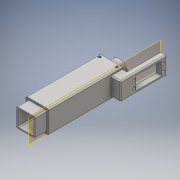
# Autodesk Inventor part: tube4
Saved by Autodesk Inventor 2016 (Build 200138000, 138)
## iProperties
Created: 2016-03-04
Part Number: tube4
Material: 一般
Document SubType Name: Modeling
Designer: Shun Hasegawa
Density: 1 g/cm^3
Appearance: 既定
Author: Shun Hasegawa
Autodesk Inventor part; units mm, degrees
ref_plane "XZ Plane" through (0, 0, 0) normal (0, 1, 0) x (-1, 0, 0)
ref_plane "XY Plane" through (0, 0, 0) normal (0, 0, 1) x (1, 0, 0)
sketch "スケッチ1" plane through (0, 0, 0) normal (0, 1, 0) x (-1, 0, 0)
  line L0 (16.5, 16.5) -> (-16.5, 16.5)
  line L1 (-16.5, 16.5) -> (-16.5, -16.5)
  line L2 (-16.5, -16.5) -> (16.5, -16.5)
  line L3 (16.5, -16.5) -> (16.5, 16.5)
  line L4 (-23.1, 0) -> (23.1, 0) projected
  line L5 (0, -23.1) -> (0, 23.1) projected
  point P0 (0, 0)
  dimension "d0" = 33
  dimension "d1" = 33
  constraints: 8 end point, 2 parallel, 1 horizontal, 1 perpendicular, 2 other
  measures "d0" distance of L2.end L0.start
  measures "d1" distance of L0.start L0.end
extrude "押し出し1" add sketch "スケッチ1" along normal blind 20
fillet "フィレット1" radius 2 4 edges at (16.5, 10, 16.5) (-16.5, 10, 16.5) (16.5, 10, -16.5) (-16.5, 10, -16.5)
sketch "スケッチ2" plane through (0, 20, 0) normal (0, 1, 0) x (1, 0, 0)
  line L0 (-20, -20) -> (20, -20)
  line L1 (20, -20) -> (20, 20)
  line L2 (20, 20) -> (-20, 20)
  line L3 (-20, 20) -> (-20, -20)
  line L4 (-14.5, -16.5) -> (14.5, -16.5) projected
  line L5 (-16.5, 14.5) -> (-16.5, -14.5) projected
  line L6 (16.5, -14.5) -> (16.5, 14.5) projected
  line L7 (14.5, 16.5) -> (-14.5, 16.5) projected
  point P0 (0, 0)
  dimension "d5" = 3.5
  dimension "d6" = 3.5
  dimension "d7" = 3.5
  dimension "d8" = 3.5
  constraints: 8 end point, 2 parallel, 1 horizontal, 1 perpendicular
  measures "d5" distance between parallel lines of L0 L4
  measures "d6" distance between parallel lines of L5 L3
  measures "d7" distance between parallel lines of L6 L1
  measures "d8" distance between parallel lines of L2 L7
extrude "押し出し2" add sketch "スケッチ2" along normal blind 30
fillet "フィレット2" radius 2 4 edges at (20, 35, 20) (20, 35, -20) (-20, 35, -20) (-20, 35, 20)
sketch "スケッチ3" plane through (0, 0, 0) normal (0, -1, 0) x (1, 0, 0)
  line L0 (12, 14) -> (-12, 14)
  line L1 (-14, 12) -> (-14, -12)
  line L2 (-12, -14) -> (12, -14)
  line L3 (14, -12) -> (14, 12)
  arc A0 (14, 12) -> (12, 14) centre (12, 12) ccw
  arc A1 (12, -14) -> (14, -12) centre (12, -12) ccw
  arc A2 (-14, -12) -> (-12, -14) centre (-12, -12) ccw
  arc A3 (-12, 14) -> (-14, 12) centre (-12, 12) ccw
  line L4 (16.5, 14.5) -> (16.5, -14.5) projected
  line L5 (14.5, -16.5) -> (-14.5, -16.5) projected
  line L6 (-14.5, 16.5) -> (14.5, 16.5) projected
  line L7 (-16.5, -14.5) -> (-16.5, 14.5) projected
  point P0 (0, 0)
  dimension "d12" = 2
  dimension "d13" = 2.5
  dimension "d14" = 2.5
  dimension "d15" = 2.5
  dimension "d16" = 2.5
  constraints: 8 end point, 8 point on circle, 8 tangent, 4 centre point, 3 equal radius, 2 parallel, 1 horizontal, 1 perpendicular
  measures "d12" radius of A0
  measures "d13" distance between parallel lines of L3 L4
  measures "d14" distance between parallel lines of L5 L2
  measures "d15" distance between parallel lines of L6 L0
  measures "d16" distance between parallel lines of L7 L1
extrude "押し出し3" cut sketch "スケッチ3" against normal up to next
sketch "スケッチ4" plane through (0, 50, 0) normal (0, 1, 0) x (1, 0, 0)
  line L0 (18, 20) -> (-18, 20) projected
  arc A0 (-18, 20) -> (-20, 18) centre (-18, 18) ccw projected
  line L1 (-20, 18) -> (-20, -18) projected
  arc A1 (-20, -18) -> (-18, -20) centre (-18, -18) ccw projected
  line L2 (-18, -20) -> (18, -20) projected
  arc A2 (18, -20) -> (20, -18) centre (18, -18) ccw projected
  line L3 (20, -18) -> (20, 18) projected
  arc A3 (20, 18) -> (18, 20) centre (18, 18) ccw projected
  line L4 (-15, 17) -> (15, 17)
  line L5 (17, 15) -> (17, -15)
  line L6 (15, -17) -> (-15, -17)
  line L7 (-17, -15) -> (-17, 15)
  arc A4 (-15, 17) -> (-17, 15) centre (-15, 15) ccw
  arc A5 (-17, -15) -> (-15, -17) centre (-15, -15) ccw
  arc A6 (15, -17) -> (17, -15) centre (15, -15) ccw
  arc A7 (17, 15) -> (15, 17) centre (15, 15) ccw
  point P0 (0, 0)
  dimension "d21" = 2
  dimension "d22" = 3
  dimension "d23" = 3
  dimension "d24" = 3
  dimension "d25" = 3
  constraints: 8 end point, 8 point on circle, 8 tangent, 4 centre point, 3 equal radius, 2 parallel, 1 horizontal, 1 perpendicular
  measures "d21" radius of A4
  measures "d22" distance between parallel lines of L7 L1
  measures "d23" distance between parallel lines of L2 L6
  measures "d24" distance between parallel lines of L3 L5
  measures "d25" distance between parallel lines of L4 L0
extrude "押し出し5" add sketch "スケッチ4" along normal blind 90
sketch "スケッチ5" plane through (0, 140, 0) normal (0, 1, 0) x (1, 0, 0)
  line L0 (18, 20) -> (-18, 20) projected
  arc A0 (-18, 20) -> (-20, 18) centre (-18, 18) ccw projected
  line L1 (-20, 18) -> (-20, -18) projected
  arc A1 (-20, -18) -> (-18, -20) centre (-18, -18) ccw projected
  line L2 (-18, -20) -> (18, -20) projected
  arc A2 (18, -20) -> (20, -18) centre (18, -18) ccw projected
  line L3 (20, -18) -> (20, 18) projected
  arc A3 (20, 18) -> (18, 20) centre (18, 18) ccw projected
  point P0 (0, 0)
extrude "押し出し6" add sketch "スケッチ5" along normal blind 10
sketch "スケッチ6" plane through (0, 150, 0) normal (0, 1, 0) x (1, 0, 0)
  circle A0 centre (0, 0) radius 15
  dimension "d30" = 30
  constraints: 1 centre point, 1 coincident
  measures "d30" diameter of A0
extrude "押し出し7" add sketch "スケッチ6" along normal blind 15
sketch "スケッチ7" plane through (0, 165, 0) normal (0, 1, 0) x (1, 0, 0)
  circle A0 centre (0, 0) radius 12
  circle A1 centre (0, 0) radius 15 projected
  dimension "d33" = 3
  constraints: 1 centre point, 1 coincident
  measures "d33" radial gap between concentric circles of A0 A1
extrude "押し出し8" cut sketch "スケッチ7" against normal up to next contours A0
sketch "スケッチ8" plane through (20, 20, 18) normal (1, 0, 0) x (0, 0, -1)
  line L0 (34, 130) -> (2, 130)
  line L1 (2, 130) -> (2, 110)
  line L2 (2, 110) -> (34, 110)
  line L3 (34, 110) -> (34, 130)
  line L4 (0, 130) -> (36, 130) projected
  line L5 (38, 0) -> (38, 130) projected
  line L6 (-2, 130) -> (-2, 0) projected
  point P0 (18, -20)
  dimension "d36" = 20
  dimension "d37" = 32
  dimension "d38" = 4
  dimension "d39" = 4
  constraints: 8 end point, 2 parallel, 1 horizontal, 1 perpendicular, 1 point on line
  measures "d36" distance of L2.end L0.start
  measures "d37" distance of L1.end L2.end
  measures "d38" distance between parallel lines of L3 L5
  measures "d39" distance between parallel lines of L6 L1
extrude "押し出し9" add sketch "スケッチ8" along normal blind 8
sketch "スケッチ9" plane through (28, 20, 18) normal (1, 0, 0) x (0, 0, -1)
  line L0 (34, 130) -> (34, 110) projected
  line L1 (34, 110) -> (2, 110)
  line L2 (2, 110) -> (2, 192)
  line L3 (2, 192) -> (34, 192)
  line L4 (34, 192) -> (34, 110)
  line L5 (34, 130) -> (2, 130) projected
  point P0 (18, -20)
  dimension "d42" = 32
  dimension "d43" = 62
  constraints: 8 end point, 2 parallel, 1 horizontal, 1 perpendicular
  measures "d42" distance of L2.end L3.end
  measures "d43" distance between parallel lines of L5 L3
extrude "押し出し10" add sketch "スケッチ9" along normal blind 9
sketch "スケッチ10" plane through (37, 20, 18) normal (1, 0, 0) x (0, 0, -1)
  line L0 (28.5, 182) -> (7.5, 182)
  line L1 (6.5, 181) -> (6.5, 138)
  line L2 (7.5, 137) -> (28.5, 137)
  line L3 (29.5, 138) -> (29.5, 181)
  line L4 (34, 192) -> (2, 192) projected
  line L5 (34, 110) -> (34, 192) projected
  line L6 (2, 192) -> (2, 110) projected
  arc A0 (29.5, 181) -> (28.5, 182) centre (28.5, 181) ccw
  arc A1 (28.5, 137) -> (29.5, 138) centre (28.5, 138) ccw
  arc A2 (6.5, 138) -> (7.5, 137) centre (7.5, 138) ccw
  arc A3 (7.5, 182) -> (6.5, 181) centre (7.5, 181) ccw
  point P0 (18, -20)
  point P1 (29.5, 182)
  point P2 (6.5, 182)
  point P3 (29.5, 137)
  dimension "d46" = 45
  dimension "d47" = 23
  dimension "d48" = 10
  dimension "d49" = 4.5
  dimension "d50" = 4.5
  dimension "d51" = 1
  constraints: 8 end point, 8 point on circle, 8 tangent, 6 point on line, 4 centre point, 3 equal radius, 2 parallel, 1 horizontal, 1 perpendicular
  measures "d46" distance of point (29.5, 137) point (29.5, 182)
  measures "d47" distance of point (29.5, 182) point (6.5, 182)
  measures "d48" distance between parallel lines of L4 L0
  measures "d49" distance between parallel lines of L3 L5
  measures "d50" distance between parallel lines of L6 L1
  measures "d51" radius of A0
extrude "押し出し11" cut sketch "スケッチ10" against normal up to next
fillet "フィレット3" radius 2 8 edges at (32.5, 212, -16) (32.5, 212, 16) (28.5, 130, -16) (28.5, 130, 16) (37, 130, 0) (37, 171, -16) (37, 171, 16) (37, 212, 0)
sketch "スケッチ11" plane through (37, 20, 18) normal (1, 0, 0) x (0, 0, -1)
  circle A0 centre (24, 185) radius 2.25
  circle A1 centre (12, 185) radius 2.25
  circle A2 centre (24, 134) radius 2.25
  circle A3 centre (12, 134) radius 2.25
  line L0 (7.5, 182) -> (28.5, 182) projected
  line L1 (28.5, 137) -> (7.5, 137) projected
  line L2 (34, 112) -> (34, 190) projected
  line L3 (2, 190) -> (2, 112) projected
  point P0 (18, -20)
  point P1 (34, 150)
  point P2 (2, 150)
  dimension "d55" = 12
  dimension "d56" = 4.5
  dimension "d57" = 4.5
  dimension "d58" = 4.5
  dimension "d59" = 4.5
  dimension "d60" = 12
  dimension "d61" = 51
  dimension "d62" = 51
  dimension "d63" = 3
  dimension "d64" = 3
  dimension "d65" = 10
  dimension "d66" = 10
  constraints: 4 centre point, 1 horizontal alignment, 1 vertical alignment
  measures "d55" distance of A1.centre A0.centre
  measures "d56" diameter of A0
  measures "d57" diameter of A1
  measures "d58" diameter of A2
  measures "d59" diameter of A3
  measures "d60" distance of A3.centre A2.centre
  measures "d61" distance of A2.centre A0.centre
  measures "d62" distance of A3.centre A1.centre
  measures "d63" distance from line of L0 A0.centre
  measures "d64" distance from line of A2.centre L1
  measures "d65" distance from line of A0.centre L2
  measures "d66" distance from line of L3 A1.centre
extrude "押し出し12" cut sketch "スケッチ11" against normal up to next contours A0
extrude "押し出し13" cut sketch "スケッチ11" against normal up to next contours A1
extrude "押し出し14" cut sketch "スケッチ11" against normal up to next contours A2
extrude "押し出し15" cut sketch "スケッチ11" against normal up to next contours A3
sketch "スケッチ21" plane through (-18, 20, 20) normal (0, 0, 1) x (1, 0, 0)
  circle A0 centre (3, 125) radius 2.25
  circle A1 centre (33, 125) radius 2.25
  line L0 (0, 0) -> (0, 130) projected
  line L1 (36, 130) -> (36, 0) projected
  line L2 (0, 130) -> (36, 130) projected
  point P0 (18, -20)
  dimension "d122" = 4.5
  dimension "d123" = 4.5
  dimension "d124" = 3
  dimension "d125" = 30
  dimension "d127" = 5
  dimension "d128" = 5
  dimension "d129" = 3
  constraints: 2 centre point
  measures "d122" diameter of A0
  measures "d123" diameter of A1
  measures "d124" distance from line of A0.centre L0
  measures "d125" distance of A1.centre A0.centre
  measures "d127" distance from line of L2 A0.centre
  measures "d128" distance from line of L2 A1.centre
  measures "d129" distance from line of L1 A1.centre
extrude "押し出し25" cut sketch "スケッチ21" against normal blind 8
ref_plane "作業平面1" through (15, 150, 0) normal (1, 0, 0) x (0, 1, 0)
sketch "スケッチ24" plane through (15, 150, 0) normal (1, 0, 0) x (0, 1, 0)
  circle A0 centre (6, 0) radius 1.5
  line L0 (-130, 20) -> (0, 20) projected
  line L1 (0, -20) -> (-130, -20) projected
  circle A1 centre (55, -6) radius 2.25 projected
  point P0 (-150, 0)
  dimension "d154" = 3
  dimension "d155" = 20
  dimension "d156" = 20
  dimension "d157" = 49
  constraints: 1 centre point
  measures "d154" diameter of A0
  measures "d155" distance from line of A0.centre L0
  measures "d156" distance from line of A0.centre L1
  measures "d157" horizontal distance of A1.centre A0.centre
extrude "押し出し29" cut sketch "スケッチ24" against normal up to surface (35 mm away) contours A0
sketch "スケッチ25" plane through (-20, 20, -18) normal (-1, 0, 0) x (0, 0, 1)
  line L0 (36, 0) -> (36, 130) projected
  line L1 (0, 0) -> (0, 130) projected
  line L2 (36, 130) -> (0, 130)
  line L3 (0, 130) -> (0, 120)
  line L4 (0, 120) -> (36, 120)
  line L5 (36, 120) -> (36, 130)
  point P0 (18, -20)
  dimension "d160" = 10
  constraints: 8 end point, 2 parallel, 1 horizontal, 1 perpendicular, 1 point on line
  measures "d160" distance between parallel lines of L4 L2
extrude "押し出し30" add sketch "スケッチ25" along normal blind 3
fillet "フィレット6" radius 3 3 edges at (-23, 145, 18) (-23, 140, 0) (-23, 145, -18)
